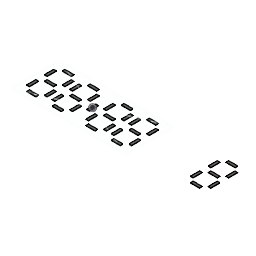
base-plate (Autodesk Fusion 360 design; units mm, degrees)
part number: 2026-01-13-11-40-15-510
Autodesk Fusion 360 part; units mm, degrees
sketch "Sketch1" plane through (0, 0, 0) normal (0, 0, 1) x (1, 0, 0)
  line L0 (16.5, 5) -> (-16.5, 5)
  line L1 (-16.5, 5) -> (-16.5, -5)
  line L2 (-16.5, -5) -> (16.5, -5)
  line L3 (16.5, -5) -> (16.5, 5)
  line L4 (16.5, 5) -> (-16.5, -5) construction
  line L5 (-16.5, 5) -> (16.5, -5) construction
  dimension "d3" = 33
  dimension "d4" = 10
  constraint horizontal L0
  constraint perpendicular L0 L1
  constraint parallel L0 L2
  constraint parallel L1 L3
  constraint coincident L4 origin
  constraint coincident L5 origin
  measures "d3" distance of L1.end L2.end
  measures "d4" distance of L0.end L1.end
extrude "Extrude1" add sketch "Sketch1" along normal blind 1 makes body 1
sketch "Sketch2" plane through (0, 0, 0) normal (0, 0, 1) x (1, 0, 0)
  line L0 (206.5, 88) -> (-206.5, 88)
  line L1 (-206.5, 88) -> (-206.5, -88)
  line L2 (-206.5, -88) -> (206.5, -88)
  line L3 (206.5, -88) -> (206.5, 88)
  line L4 (206.5, 88) -> (-206.5, -88) construction
  line L5 (-206.5, 88) -> (206.5, -88) construction
  dimension "d9" = 413
  dimension "d10" = 176
  constraint horizontal L0
  constraint perpendicular L0 L1
  constraint parallel L0 L2
  constraint parallel L1 L3
  constraint coincident L4 origin
  constraint coincident L5 origin
  measures "d9" distance of L1.end L2.end
  measures "d10" distance of L0.end L1.end
move_body "Move1" bodies 1 to x (1, 0, 0) y (0, 1, 0) z (0, 0, 1) at (140, 0, 0)
sketch "Sketch3" plane through (0, 0, 0) normal (0, 0, 1) x (1, 0, 0)
  line L0 (125, -35) -> (135, -35)
  line L1 (135, -35) -> (135, -2)
  line L2 (135, -2) -> (125, -2)
  line L3 (125, -2) -> (125, -35)
  dimension "d11" = 10
  dimension "d12" = 33
  constraint horizontal L0
  constraint vertical L1
  constraint horizontal L2
  constraint vertical L3
  measures "d11" distance of L0.start L0.end
  measures "d12" distance of L0.start L2.end
extrude "Extrude2" add sketch "Sketch3" along normal blind 1 separate body makes body 2
move_body "Move8" bodies 2 to x (1, 0, 0) y (0, 1, 0) z (0, 0, 1) at (10, -10, 0)
move_body "Move10" bodies 2 to x (1, 0, 0) y (0, 1, 0) z (0, 0, 1) at (-25, 7, 0)
move_body "Move11" bodies 1 to x (1, 0, 0) y (0, 1, 0) z (0, 0, 1) at (-3.5, 30, 0)
move_body "Move12" bodies 1 to x (1, 0, 0) y (0, 1, 0) z (0, 0, 1) at (30, 0, 0)
copy_body "CopyPasteBodies6" bodies 2 makes body 3
move_body "Move13" bodies 3 to x (1, 0, 0) y (0, 1, 0) z (0, 0, 1) at (103, 0, 0)
copy_body "CopyPasteBodies7" bodies 1 makes body 4
move_body "Move14" bodies 4 to x (1, 0, 0) y (0, 1, 0) z (0, 0, 1) at (0, -103, 0)
copy_body "CopyPasteBodies8" bodies 2 makes body 5
move_body "Move15" bodies 5 to x (1, 0, 0) y (0, 1, 0) z (0, 0, 1) at (0, 103, 0)
copy_body "CopyPasteBodies9" bodies 3 makes body 6
move_body "Move16" bodies 6 to x (1, 0, 0) y (0, 1, 0) z (0, 0, 1) at (0, 103, 0)
copy_body "CopyPasteBodies10" bodies 1 makes body 7
move_body "Move17" bodies 7 to x (1, 0, 0) y (0, 1, 0) z (0, 0, 1) at (0, 103, 0)
move_body "Move18" bodies 4 to x (1, 0, 0) y (0, 1, 0) z (0, 0, 1) at (-20, 10, 0)
move_body "Move19" bodies 3 to x (1, 0, 0) y (0, 1, 0) z (0, 0, 1) at (-40, 0, 0)
move_body "Move20" bodies 1 to x (1, 0, 0) y (0, 1, 0) z (0, 0, 1) at (-20, -10, 0)
move_body "Move21" bodies 5 to x (1, 0, 0) y (0, 1, 0) z (0, 0, 1) at (0, -20, 0)
move_body "Move22" bodies 6 to x (1, 0, 0) y (0, 1, 0) z (0, 0, 1) at (-40, -20, 0)
move_body "Move23" bodies 7 to x (1, 0, 0) y (0, 1, 0) z (0, 0, 1) at (-20, -30, 0)
move_body "Move24" bodies 7 to x (1, 0, 0) y (0, 1, 0) z (0, 0, 1) at (10, 0, 0)
move_body "Move25" bodies 6 to x (1, 0, 0) y (0, 1, 0) z (0, 0, 1) at (20, 0, 0)
move_body "Move26" bodies 1 to x (1, 0, 0) y (0, 1, 0) z (0, 0, 1) at (10, 0, 0)
move_body "Move27" bodies 3 to x (1, 0, 0) y (0, 1, 0) z (0, 0, 1) at (20, 0, 0)
move_body "Move28" bodies 4 to x (1, 0, 0) y (0, 1, 0) z (0, 0, 1) at (10, 0, 0)
move_body "Move29" bodies 1 2 4 6 3 7 5 to x (1, 0, 0) y (0, 1, 0) z (0, 0, 1) at (275, 0, 0)
move_body "Move34" bodies 1 to x (1, 0, 0) y (0, 1, 0) z (0, 0, 1) at (-10, -10, 0)
move_body "Move35" bodies 3 to x (1, 0, 0) y (0, 1, 0) z (0, 0, 1) at (-20, 0, 0)
move_body "Move36" bodies 4 to x (1, 0, 0) y (0, 1, 0) z (0, 0, 1) at (-10, 10, 0)
move_body "Move37" bodies 5 to x (1, 0, 0) y (0, 1, 0) z (0, 0, 1) at (0, -20, 0)
move_body "Move38" bodies 6 to x (1, 0, 0) y (0, 1, 0) z (0, 0, 1) at (-20, -20, 0)
move_body "Move39" bodies 7 to x (1, 0, 0) y (0, 1, 0) z (0, 0, 1) at (-10, -30, 0)
copy_body "CopyPasteBodies15" bodies 1 2 3 4 5 6 7 makes body 8 makes body 9 makes body 10 makes body 11 makes body 12 makes body 13 makes body 14
move_body "Move40" bodies 8 9 10 11 12 13 14 to x (1, 0, 0) y (0, 1, 0) z (0, 0, 1) at (-600, 0, 0)
copy_body "CopyPasteBodies16" bodies 8 9 10 11 12 13 14 makes body 15 makes body 16 makes body 17 makes body 18 makes body 19 makes body 20 makes body 21
move_body "Move41" bodies 15 16 17 18 19 20 21 to x (1, 0, 0) y (0, 1, 0) z (0, 0, 1) at (90, 0, 0)
copy_body "CopyPasteBodies17" bodies 8 9 10 11 12 13 14 makes body 22 makes body 23 makes body 24 makes body 25 makes body 26 makes body 27 makes body 28
move_body "Move42" bodies 22 23 24 25 26 27 28 to x (1, 0, 0) y (0, 1, 0) z (0, 0, 1) at (210, 0, 0)
copy_body "CopyPasteBodies18" bodies 8 9 10 11 12 13 14 makes body 29 makes body 30 makes body 31 makes body 32 makes body 33 makes body 34 makes body 35
move_body "Move43" bodies 29 30 31 32 33 34 35 to x (1, 0, 0) y (0, 1, 0) z (0, 0, 1) at (300, 0, 0)
copy_body "CopyPasteBodies19" bodies 5 makes body 36
move_body "Move44" bodies 36 to x (1, 0, 0) y (0, 1, 0) z (0, 0, 1) at (-418.5, -31.5, 0)
move_body "Move45" bodies 28 25 27 26 24 23 22 29 30 31 32 33 34 35 36 21 19 20 18 17 16 15 14 13 12 11 10 9 8 to x (1, 0, 0) y (0, 1, 0) z (0, 0, 1) at (28.4792, -10.017, 0)
equation "LED_WIDTH = 33 mm"
equation "LED_HEIGHT = 10 mm"
equation "d3 = LED_WIDTH"
equation "d4 = LED_HEIGHT"
equation "BOARD_WIDTH = 413 mm"
equation "BOARD_HEIGHT = 176 mm"
equation "d9 = BOARD_WIDTH"
equation "d10 = BOARD_HEIGHT"
equation "d11 = LED_HEIGHT"
equation "d12 = LED_WIDTH"
